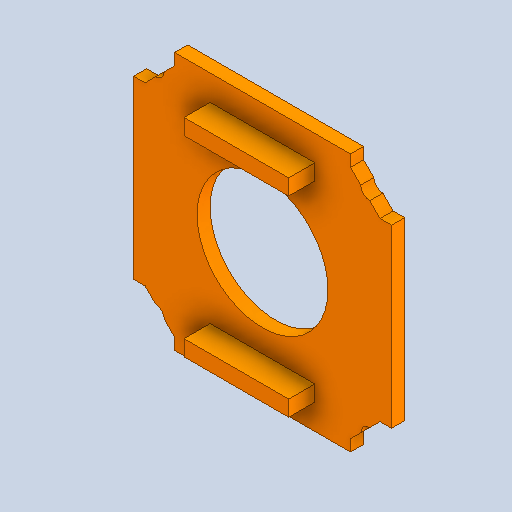
# Autodesk Inventor part: Sample Holder
Saved by Autodesk Inventor 2023 (Build 270158030, 158C)
## iProperties
Created: 2021-10-06
Part Number: Sample Holder
Material: Generic
Document SubType Name: Modeling
Designer: user
Density: 1 g/cm^3
Appearance: Plastic Orange
Author: user
Autodesk Inventor part; units mm, degrees
ref_plane "YZ Plane" through (0, 0, 0) normal (1, 0, 0) x (0, 1, 0)
sketch "Sketch1" plane through (0, 0, 0) normal (0, 0, 1) x (1, 0, 0)
  line L0 (-17.9, 11.25) -> (-21.066, 11.25) projected
  line L1 (-17.9, 14.6269) -> (-17.9, 11.25) projected
  line L2 (-14.6269, 17.9) -> (-17.9, 14.6269) projected
  line L3 (14.6269, 17.9) -> (-14.6269, 17.9) projected
  line L4 (17.9, 14.6269) -> (14.6269, 17.9) projected
  line L5 (17.9, 11.25) -> (17.9, 14.6269) projected
  line L6 (21.066, 11.25) -> (17.9, 11.25) projected
  line L7 (21.066, 11.25) -> (21.066, -11.25) projected
  line L8 (17.9, -11.25) -> (21.066, -11.25) projected
  line L9 (17.9, -14.6269) -> (17.9, -11.25) projected
  line L10 (14.6269, -17.9) -> (17.9, -14.6269) projected
  line L11 (-14.6269, -17.9) -> (14.6269, -17.9) projected
  line L12 (-17.9, -14.6269) -> (-14.6269, -17.9) projected
  line L13 (-17.9, -11.25) -> (-17.9, -14.6269) projected
  line L14 (-21.066, -11.25) -> (-17.9, -11.25) projected
  line L15 (-21.066, 11.25) -> (-21.066, -11.25) projected
  circle A0 centre (-20.8, 14.4) radius 2.35 projected
  circle A1 centre (20.8, -14.4) radius 2.35 projected
  circle A2 centre (20.8, 14.4) radius 2.35 projected
  circle A3 centre (-20.8, -14.4) radius 2.35 projected
  line L16 (17.05, -24.9) -> (-17.05, -24.9) projected
  line L17 (17.05, -22.55) -> (17.05, -24.9) projected
  line L18 (19.0152, -20.5848) -> (17.05, -22.55) projected
  arc A4 (20.5848, -19.0152) -> (19.0152, -20.5848) centre (20.5135, -20.5135) ccw projected
  line L19 (22.55, -17.05) -> (20.5848, -19.0152) projected
  line L20 (24.9, -17.05) -> (22.55, -17.05) projected
  line L21 (24.9, 17.05) -> (24.9, -17.05) projected
  line L22 (22.55, 17.05) -> (24.9, 17.05) projected
  line L23 (20.5848, 19.0152) -> (22.55, 17.05) projected
  arc A5 (19.0152, 20.5848) -> (20.5848, 19.0152) centre (20.5135, 20.5135) ccw projected
  line L24 (17.05, 22.55) -> (19.0152, 20.5848) projected
  line L25 (17.05, 24.9) -> (17.05, 22.55) projected
  line L26 (-17.05, 24.9) -> (17.05, 24.9) projected
  line L27 (-17.05, 22.55) -> (-17.05, 24.9) projected
  line L28 (-19.0152, 20.5848) -> (-17.05, 22.55) projected
  arc A6 (-20.5848, 19.0152) -> (-19.0152, 20.5848) centre (-20.5135, 20.5135) ccw projected
  line L29 (-22.55, 17.05) -> (-20.5848, 19.0152) projected
  line L30 (-24.9, 17.05) -> (-22.55, 17.05) projected
  line L31 (-24.9, -17.05) -> (-24.9, 17.05) projected
  line L32 (-22.55, -17.05) -> (-24.9, -17.05) projected
  line L33 (-20.5848, -19.0152) -> (-22.55, -17.05) projected
  arc A7 (-19.0152, -20.5848) -> (-20.5848, -19.0152) centre (-20.5135, -20.5135) ccw projected
  line L34 (-17.05, -22.55) -> (-19.0152, -20.5848) projected
  line L35 (-17.05, -24.9) -> (-17.05, -22.55) projected
  line L36 (24.65, -16.8) -> (22.4464, -16.8)
  line L37 (22.4464, -16.8) -> (20.4827, -18.7637)
  arc A8 (20.4827, -18.7637) -> (18.7637, -20.4827) centre (20.5135, -20.5135) ccw
  line L38 (18.7637, -20.4827) -> (16.8, -22.4464)
  line L39 (16.8, -22.4464) -> (16.8, -24.65)
  line L40 (16.8, -24.65) -> (-16.8, -24.65)
  line L41 (-16.8, -24.65) -> (-16.8, -22.4464)
  line L42 (-16.8, -22.4464) -> (-18.7637, -20.4827)
  arc A9 (-18.7637, -20.4827) -> (-20.4827, -18.7637) centre (-20.5135, -20.5135) ccw
  line L43 (-20.4827, -18.7637) -> (-22.4464, -16.8)
  line L44 (-22.4464, -16.8) -> (-24.65, -16.8)
  line L45 (-24.65, -16.8) -> (-24.65, 16.8)
  line L46 (-24.65, 16.8) -> (-22.4464, 16.8)
  line L47 (-22.4464, 16.8) -> (-20.4827, 18.7637)
  arc A10 (-20.4827, 18.7637) -> (-18.7637, 20.4827) centre (-20.5135, 20.5135) ccw
  line L48 (-18.7637, 20.4827) -> (-16.8, 22.4464)
  line L49 (-16.8, 22.4464) -> (-16.8, 24.65)
  line L50 (-16.8, 24.65) -> (16.8, 24.65)
  line L51 (16.8, 24.65) -> (16.8, 22.4464)
  line L52 (16.8, 22.4464) -> (18.7637, 20.4827)
  arc A11 (18.7637, 20.4827) -> (20.4827, 18.7637) centre (20.5135, 20.5135) ccw
  line L53 (20.4827, 18.7637) -> (22.4464, 16.8)
  line L54 (22.4464, 16.8) -> (24.65, 16.8)
  line L55 (24.65, 16.8) -> (24.65, -16.8)
  circle A12 centre (0, 0) radius 12.5
  line L56 (22.4464, 16.8) -> (-22.4464, 16.8)
  line L57 (-22.4464, -16.8) -> (22.4464, -16.8)
  line L58 (-10, -15.3) -> (10, -15.3)
  line L59 (10, -15.3) -> (10, -18.3)
  line L60 (10, -18.3) -> (-10, -18.3)
  line L61 (-10, -18.3) -> (-10, -15.3)
  line L62 (-10, -15.3) -> (10, -18.3) construction
  line L63 (10, -15.3) -> (-10, -18.3) construction
  line L64 (-10, 18.3) -> (10, 18.3)
  line L65 (10, 18.3) -> (10, 15.3)
  line L66 (10, 15.3) -> (-10, 15.3)
  line L67 (-10, 15.3) -> (-10, 18.3)
  line L68 (-10, 18.3) -> (10, 15.3) construction
  line L69 (10, 18.3) -> (-10, 15.3) construction
  line L70 (-10, 19.8) -> (10, 19.8)
  line L71 (10, 19.8) -> (10, 16.8)
  line L72 (10, 16.8) -> (-10, 16.8)
  line L73 (-10, 16.8) -> (-10, 19.8)
  line L74 (-10, 19.8) -> (10, 16.8) construction
  line L75 (10, 19.8) -> (-10, 16.8) construction
  line L76 (-10, -16.8) -> (10, -16.8)
  line L77 (10, -16.8) -> (10, -19.8)
  line L78 (10, -19.8) -> (-10, -19.8)
  line L79 (-10, -19.8) -> (-10, -16.8)
  line L80 (-10, -16.8) -> (10, -19.8) construction
  line L81 (10, -16.8) -> (-10, -19.8) construction
  point P0 (0, -16.8)
  point P1 (0, 16.8)
  point P2 (0, 18.3)
  point P3 (0, -18.3)
  dimension "d0" = 0.25
  dimension "d1" = 25
  dimension "d2" = 20
  dimension "d3" = 3
  dimension "d4" = 20
  dimension "d5" = 3
  dimension "d6" = 20
  dimension "d7" = 3
  dimension "d8" = 20
  dimension "d9" = 3
  constraints: 92 end point, 12 midpoint, 9 parallel, 8 point on circle, 5 centre point, 5 horizontal, 4 perpendicular, 1 coincident, 23 other
  measures "d0" distance between parallel lines of L21 L55
  measures "d1" diameter of A12
  measures "d2" distance of L59.end L60.end
  measures "d3" distance of L58.end L59.end
  measures "d4" distance of L65.end L66.end
  measures "d5" distance of L64.end L65.end
  measures "d6" distance of L71.end L72.end
  measures "d7" distance of L70.end L71.end
  measures "d8" distance of L77.end L78.end
  measures "d9" distance of L76.end L77.end
ref_plane "Work Plane1" through (-24.9, -24.9, 7.7) normal (0, 0, 1) x (1, 0, 0)
extrude "Extrusion1" add sketch "Sketch1" along normal blind 2.5 from surface at 7.7 contours L1 L2 L56 L67 L66 L65 L4 L5 L6 L7 L8 L9 L10 L57 L59 L58 L61 L12 L13 L14 L15 L0 | L0 L15 L14 L13 L12 L57 L44 L45 L46 L56 L2 L1 | L56 L47 A10 L48 L49 L50 L51 L52 A11 L53 L4 L3 L65 L71 L70 L73 L67 L2 | L2 L3 L67 L56 | L67 L3 L65 L56 | L56 L65 L66 L67 | L67 L64 L65 L3 | L65 L3 L4 L56 | L57 L61 L11 L12 | L12 L11 L61 L79 L78 L77 L59 L10 L57 L37 A8 L38 L39 L40 L41 L42 A9 L43 | L73 L70 L71 L64 | L56 L54 L55 L36 L57 L10 L9 L8 L7 L6 L5 L4 | L61 L58 L59 L57 | L57 L59 L11 L61 | L11 L59 L60 L61 | L57 L10 L11 L59 | L60 L77 L78 L79 | A0 | A1 | A2 | A3
sketch "Sketch2" plane through (0, 0, 0) normal (0, 0, 1) x (1, 0, 0)
  line L0 (-17.9, 11.25) -> (-21.066, 11.25)
  line L1 (-17.9, 14.6269) -> (-17.9, 11.25)
  line L2 (-14.6269, 17.9) -> (-17.9, 14.6269)
  line L3 (14.6269, 17.9) -> (-14.6269, 17.9)
  line L4 (17.9, 14.6269) -> (14.6269, 17.9)
  line L5 (17.9, 11.25) -> (17.9, 14.6269)
  line L6 (21.066, 11.25) -> (17.9, 11.25)
  line L7 (21.066, 11.25) -> (21.066, -11.25)
  line L8 (17.9, -11.25) -> (21.066, -11.25)
  line L9 (17.9, -14.6269) -> (17.9, -11.25)
  line L10 (14.6269, -17.9) -> (17.9, -14.6269)
  line L11 (-14.6269, -17.9) -> (14.6269, -17.9)
  line L12 (-17.9, -14.6269) -> (-14.6269, -17.9)
  line L13 (-17.9, -11.25) -> (-17.9, -14.6269)
  line L14 (-21.066, -11.25) -> (-17.9, -11.25)
  line L15 (-21.066, 11.25) -> (-21.066, -11.25)
  circle A0 centre (-20.8, 14.4) radius 2.35
  circle A1 centre (20.8, -14.4) radius 2.35
  circle A2 centre (20.8, 14.4) radius 2.35
  circle A3 centre (-20.8, -14.4) radius 2.35
  line L16 (17.05, -24.9) -> (-17.05, -24.9)
  line L17 (17.05, -22.55) -> (17.05, -24.9)
  line L18 (19.0152, -20.5848) -> (17.05, -22.55)
  arc A4 (20.5848, -19.0152) -> (19.0152, -20.5848) centre (20.5135, -20.5135) ccw
  line L19 (22.55, -17.05) -> (20.5848, -19.0152)
  line L20 (24.9, -17.05) -> (22.55, -17.05)
  line L21 (24.9, 17.05) -> (24.9, -17.05)
  line L22 (22.55, 17.05) -> (24.9, 17.05)
  line L23 (20.5848, 19.0152) -> (22.55, 17.05)
  arc A5 (19.0152, 20.5848) -> (20.5848, 19.0152) centre (20.5135, 20.5135) ccw
  line L24 (17.05, 22.55) -> (19.0152, 20.5848)
  line L25 (17.05, 24.9) -> (17.05, 22.55)
  line L26 (-17.05, 24.9) -> (17.05, 24.9)
  line L27 (-17.05, 22.55) -> (-17.05, 24.9)
  line L28 (-19.0152, 20.5848) -> (-17.05, 22.55)
  arc A6 (-20.5848, 19.0152) -> (-19.0152, 20.5848) centre (-20.5135, 20.5135) ccw
  line L29 (-22.55, 17.05) -> (-20.5848, 19.0152)
  line L30 (-24.9, 17.05) -> (-22.55, 17.05)
  line L31 (-24.9, -17.05) -> (-24.9, 17.05)
  line L32 (-22.55, -17.05) -> (-24.9, -17.05)
  line L33 (-20.5848, -19.0152) -> (-22.55, -17.05)
  arc A7 (-19.0152, -20.5848) -> (-20.5848, -19.0152) centre (-20.5135, -20.5135) ccw
  line L34 (-17.05, -22.55) -> (-19.0152, -20.5848)
  line L35 (-17.05, -24.9) -> (-17.05, -22.55)
  line L36 (24.65, -16.8) -> (22.4464, -16.8)
  line L37 (22.4464, -16.8) -> (20.4827, -18.7637)
  arc A8 (20.4827, -18.7637) -> (18.7637, -20.4827) centre (20.5135, -20.5135) ccw
  line L38 (18.7637, -20.4827) -> (16.8, -22.4464)
  line L39 (16.8, -22.4464) -> (16.8, -24.65)
  line L40 (16.8, -24.65) -> (-16.8, -24.65)
  line L41 (-16.8, -24.65) -> (-16.8, -22.4464)
  line L42 (-16.8, -22.4464) -> (-18.7637, -20.4827)
  arc A9 (-18.7637, -20.4827) -> (-20.4827, -18.7637) centre (-20.5135, -20.5135) ccw
  line L43 (-20.4827, -18.7637) -> (-22.4464, -16.8)
  line L44 (-22.4464, -16.8) -> (-24.65, -16.8)
  line L45 (-24.65, -16.8) -> (-24.65, 16.8)
  line L46 (-24.65, 16.8) -> (-22.4464, 16.8)
  line L47 (-22.4464, 16.8) -> (-20.4827, 18.7637)
  arc A10 (-20.4827, 18.7637) -> (-18.7637, 20.4827) centre (-20.5135, 20.5135) ccw
  line L48 (-18.7637, 20.4827) -> (-16.8, 22.4464)
  line L49 (-16.8, 22.4464) -> (-16.8, 24.65)
  line L50 (-16.8, 24.65) -> (16.8, 24.65)
  line L51 (16.8, 24.65) -> (16.8, 22.4464)
  line L52 (16.8, 22.4464) -> (18.7637, 20.4827)
  arc A11 (18.7637, 20.4827) -> (20.4827, 18.7637) centre (20.5135, 20.5135) ccw
  line L53 (20.4827, 18.7637) -> (22.4464, 16.8)
  line L54 (22.4464, 16.8) -> (24.65, 16.8)
  line L55 (24.65, 16.8) -> (24.65, -16.8)
  circle A12 centre (0, 0) radius 12.5
  line L56 (22.4464, 16.8) -> (-22.4464, 16.8)
  line L57 (-22.4464, -16.8) -> (22.4464, -16.8)
  line L58 (-10, -15.3) -> (10, -15.3)
  line L59 (10, -15.3) -> (10, -18.3)
  line L60 (10, -18.3) -> (-10, -18.3)
  line L61 (-10, -18.3) -> (-10, -15.3)
  line L62 (-10, -15.3) -> (10, -18.3) construction
  line L63 (10, -15.3) -> (-10, -18.3) construction
  line L64 (-10, 18.3) -> (10, 18.3)
  line L65 (10, 18.3) -> (10, 15.3)
  line L66 (10, 15.3) -> (-10, 15.3)
  line L67 (-10, 15.3) -> (-10, 18.3)
  line L68 (-10, 18.3) -> (10, 15.3) construction
  line L69 (10, 18.3) -> (-10, 15.3) construction
  line L70 (-10, 19.8) -> (10, 19.8)
  line L71 (10, 19.8) -> (10, 16.8)
  line L72 (10, 16.8) -> (-10, 16.8)
  line L73 (-10, 16.8) -> (-10, 19.8)
  line L74 (-10, 19.8) -> (10, 16.8) construction
  line L75 (10, 19.8) -> (-10, 16.8) construction
  line L76 (-10, -16.8) -> (10, -16.8)
  line L77 (10, -16.8) -> (10, -19.8)
  line L78 (10, -19.8) -> (-10, -19.8)
  line L79 (-10, -19.8) -> (-10, -16.8)
  line L80 (-10, -16.8) -> (10, -19.8) construction
  line L81 (10, -16.8) -> (-10, -19.8) construction
  point P0 (0, -16.8)
  point P1 (0, 16.8)
  point P2 (0, 18.3)
  point P3 (0, -18.3)
  point P4 (10, -16.8)
  point P5 (-10, -16.8)
  point P6 (-10, 16.8)
  point P7 (10, 16.8)
  dimension "d1" = 25
  dimension "d12" = 0.25
  dimension "d13" = 25
  dimension "d14" = 20
  dimension "d15" = 3
  dimension "d16" = 20
  dimension "d17" = 3
  dimension "d18" = 20
  dimension "d19" = 3
  dimension "d20" = 20
  dimension "d21" = 3
  constraints: 164 end point, 16 point on circle, 13 centre point, 12 midpoint, 9 parallel, 5 horizontal, 4 perpendicular, 1 coincident, 23 other
  measures "d12" distance between parallel lines of L21 L55
  measures "d13" diameter of A12
  measures "d14" distance of L59.end L60.end
  measures "d15" distance of L58.end L59.end
  measures "d16" distance of L65.end L66.end
  measures "d17" distance of L64.end L65.end
  measures "d18" distance of L71.end L72.end
  measures "d19" distance of L70.end L71.end
  measures "d20" distance of L77.end L78.end
  measures "d21" distance of L76.end L77.end
extrude "Extrusion2" add sketch "Sketch2" along normal blind 5 from surface at 10.2 contours L67 L3 L65 L56 | L67 L64 L65 L3 | L73 L70 L71 L64 | L57 L59 L11 L61 | L11 L59 L60 L61 | L60 L77 L78 L79
sketch "Sketch3" plane through (-16.8, 24.65, 10.2) normal (0, 1, 0) x (1, 0, 0)
  circle A0 centre (-3.1, -24.6) radius 2.0625 projected
  circle A1 centre (36.7, -24.6) radius 2.0625 projected
  circle A2 centre (36.7, -4.8) radius 2.0625 projected
  circle A3 centre (-3.1, -4.8) radius 2.0625 projected
  circle A4 centre (26.8, 6.35) radius 1.5625 projected
  circle A5 centre (6.8, 6.35) radius 1.5625 projected
  line L0 (-6.1, -31.9) -> (-6.1, 10.2) projected
  line L1 (-6.1, -31.9) -> (-0.25, -31.9) projected
  line L2 (-0.25, -31.9) -> (-0.25, 2.5) projected
  line L3 (-0.25, 2.5) -> (33.85, 2.5) projected
  line L4 (33.85, 2.5) -> (33.85, -31.9) projected
  line L5 (33.85, -31.9) -> (39.7, -31.9) projected
  line L6 (39.7, 10.2) -> (39.7, -31.9) projected
  line L7 (39.7, 10.2) -> (-6.1, 10.2) projected
  line L8 (28.447, 2.5) -> (5.153, 2.5)
  point P0 (16.8, 10.2)
  constraints: 2 end point, 1 horizontal
ref_plane "Work Plane2" through (-22.9, -24.9, 0) normal (0, -1, 0) x (1, 0, 0)
extrude "Extrusion3" [suppressed]
pattern_circular "Circular Pattern1" [suppressed]
body "Solid1"
